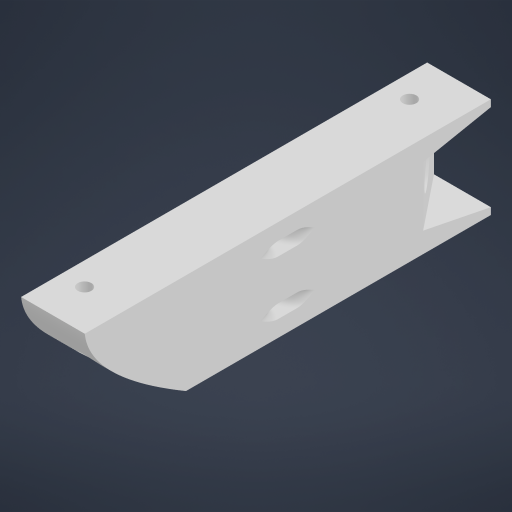
# Autodesk Inventor part: flank
Saved by Autodesk Inventor 2024 (Build 280153000, 153)
## iProperties
Created: 2024-06-07
Part Number: flank
Material: Generic
Document SubType Name: Modeling
Designer: markm
Density: 1 g/cm^3
Appearance: Default
Author: markm
Autodesk Inventor part; units mm, degrees
ref_plane "YZ Plane" through (0, 0, 0) normal (1, 0, 0) x (0, 1, 0)
ref_plane "XZ Plane" through (0, 0, 0) normal (0, 1, 0) x (-1, 0, 0)
sketch "Sketch3" plane through (0, 0, 0) normal (1, 0, 0) x (0, 1, 0)
  line L0 (20, 0) -> (-20, 0)
  line L1 (-20, 0) -> (-20, 150) construction
  line L2 (-20, 150) -> (20, 150) construction
  line L3 (20, 150) -> (20, 0) construction
  line L4 (20, 150) -> (3.094, 150) construction
  line L5 (3.094, 150) -> (-20, 110) construction
  spline S0 degree 2 poles (20, 150) (3.094, 150) (-20, 110) knots 1 1 1 2 2 2
  line L6 (18.5, 149.9225) -> (18.5, 0)
  line L7 (-18.5, 0) -> (-18.5, 112.5669)
  line L8 (0, 0) -> (0, 119.3226) construction
  line L9 (18.5, 0) -> (18.5, 10) construction
  line L10 (18.5, 10) -> (0, 10) construction
  spline S1 degree 2 poles (18.5, 0) (18.5, 10) (0, 10) knots 1 1 1 2 2 2
  line L11 (0, 15) -> (15.8455, 15) construction
  line L12 (-18.5, 0) -> (-18.5, 10) construction
  line L13 (-18.5, 10) -> (0, 10) construction
  spline S2 degree 2 poles (-18.5, 0) (-18.5, 10) (0, 10) knots 1 1 1 2 2 2
  line L14 (16, 0) -> (11, 25)
  line L15 (11, 25) -> (-11, 25)
  line L16 (-11, 25) -> (-16, 0)
  arc A0 (11, 25) -> (-11, 25) centre (0, 22.8) ccw
  dimension "d14" = 40
  dimension "d15" = 150
  dimension "d16" = 40
  dimension "d17" = 30
  dimension "d18" = 1.5
  dimension "d47" = 15
  dimension "d48" = 5
  dimension "d50" = 5
  dimension "d51" = 25
  dimension "d52" = 2.5
  constraints: 22 end point, 9 point on line, 4 perpendicular, 3 horizontal, 3 parallel, 2 point on circle, 1 centre point, 1 coincident, 1 midpoint, 1 symmetric about line, 1 tangent, 13 other
  measures "d14" distance between parallel lines of L1 L3
  measures "d15" distance of L2.end L0.start
  measures "d16" vertical distance of L4.end L5.end
  measures "d17" angle of L1 L5
  measures "d18" distance between parallel lines of L3 L6
  measures "d47" distance between parallel lines of L0 L11
  measures "d48" distance between parallel lines of L11 L10
  measures "d50" horizontal distance of L14.start L14.end
  measures "d51" vertical distance of L14.start L14.end
  measures "d52" distance of L6.end L14.start
extrude "Extrusion3" add sketch "Sketch3" along normal blind 15 and the other way blind 8.5 contours S1 L14 A0 L16 S2 L7 S0 L6 | L0 L14 S1 | L0 S2 L16 | L15 A0
sketch "Sketch4" plane through (-8.5, 18.5, 149.9225) normal (0, 1, 0) x (1, 0, 0)
  line L0 (8.5, 149.9225) -> (8.5, 14.9225) construction
  circle A0 centre (8.5, 14.9225) radius 2.5
  circle A1 centre (8.5, 134.9225) radius 2.5
  line L1 (23.5, 149.9225) -> (23.5, 0) projected
  line L2 (0, 149.9225) -> (23.5, 149.9225) projected
  line L3 (0, 149.9225) -> (11.9483, 138.5432)
  arc A2 (13.5, 134.9225) -> (11.9483, 138.5432) centre (8.5, 134.9225) ccw
  line L4 (13.5, 134.9225) -> (13.5, 99.9225)
  line L5 (13.5, 99.9225) -> (0, 99.9225)
  line L6 (0, 99.9225) -> (0, 149.9225)
  line L7 (2.5, 149.9225) -> (2.5, 99.9225)
  line L8 (0, 0) -> (0, 149.9225) projected
  line L9 (23.5, 124.9225) -> (0, 124.9225)
  line L10 (2.5, 149.9225) -> (23.5, 124.9225)
  point P0 (33.5, 149.9225)
  point P1 (0, 124.9225)
  dimension "d23" = 5
  dimension "d24" = 120
  dimension "d25" = 15
  dimension "d36" = 10
  dimension "d40" = 5
  dimension "d54" = 50
  dimension "d57" = 2.5
  constraints: 16 end point, 5 point on line, 3 centre point, 3 perpendicular, 3 vertical, 2 point on circle, 2 tangent, 1 coincident, 1 concentric, 1 equal radius
  measures "d23" diameter of A0
  measures "d24" distance of A1.centre L0.end
  measures "d25" distance of A1.centre L0.start
  measures "d36" distance of L1.start point (33.5, 149.923)
  measures "d40" radius of A2
  measures "d54" distance between parallel lines of L2 L5
  measures "d57" distance between parallel lines of L6 L7
extrude "Extrusion8" add sketch "Sketch4" against normal up to surface (37 mm away) contours A1 | L9 L4 A2 L3 L7 L10 | L7 L3 L2 | L9 L7 L3 A2 L4 | L3 L7 L9 L6
extrude "Extrusion4" cut sketch "Sketch4" against normal blind 16 contours A0 | A1
sketch "Sketch5" plane through (-8.5, -18.5, 0) normal (0, -1, 0) x (1, 0, 0)
  line L0 (8.5, 0) -> (8.5, 95) construction
  circle A0 centre (8.5, 95) radius 2.5
  circle A1 centre (8.5, 15) radius 2.5
  dimension "d58" = 5
  dimension "d59" = 95
  dimension "d60" = 15
  constraints: 2 centre point, 2 end point, 1 coincident, 1 equal radius, 1 point on line, 1 vertical
  measures "d58" diameter of A1
  measures "d59" distance of L0.start L0.end
  measures "d60" distance of L0.start A1.centre
extrude "Extrusion9" cut sketch "Sketch5" against normal blind 16
sketch "Sketch6" plane through (0, 0, 0) normal (0, 0, 1) x (1, 0, 0)
  arc A0 (3.5291, 0.4815) -> (11.4709, 0.4815) centre (7.5, 0) ccw construction
  circle A1 centre (7.5, 0) radius 5
  line L0 (15, -11) -> (15, 11) construction
  line L1 (15, 0) -> (7.5, 0) construction
  point P0 (0, 0)
  dimension "d63" = 10
  dimension "d69" = 7.5
  constraints: 2 centre point, 2 coincident, 2 end point, 2 point on circle, 1 horizontal, 1 midpoint
  measures "d63" diameter of A1
  measures "d69" distance of L1.start L1.end
extrude "Extrusion10" cut sketch "Sketch6" along normal through all
thicken "Thicken1" [suppressed]
ref_plane "Work Plane1" through (0, 0, 75) normal (0, 0, 1) x (1, 0, 0)
sketch "Sketch8" plane through (0, 0, 75) normal (0, 0, 1) x (1, 0, 0)
  circle A0 centre (7.5, 0) radius 5 construction
  line L0 (-8.5, -18.5) -> (-8.5, 18.5) construction
  line L1 (-8.5, 18.5) -> (15, 18.5) construction
  line L2 (15, 18.5) -> (15, -18.5) construction
  line L3 (15, -18.5) -> (-8.5, -18.5) construction
  line L4 (15, 10) -> (7.5, 10)
  line L5 (-2.5, 0) -> (-2.5, 0)
  line L6 (-2.5, 0) -> (15, 0) construction
  arc A1 (7.5, 10) -> (-2.5, 0) centre (7.5, 0) ccw
  point P0 (0, 0)
  point P1 (-2.5, 10)
  dimension "d71" = 10
  dimension "d72" = 17.5
  dimension "d73" = 10
  constraints: 6 end point, 3 point on line, 2 perpendicular, 2 point on circle, 2 tangent, 1 centre point, 1 horizontal, 1 midpoint
  measures "d71" distance between parallel lines of L6 L4
  measures "d72" distance of L4.start point (-2.5, 10)
  measures "d73" radius of A1
sketch "Sketch9" plane through (15, 0, 0) normal (1, 0, 0) x (0, 0, -1)
  circle A0 centre (-75, 10) radius 2.5
  point P0 (0, 0)
  dimension "d74" = 5
  constraints: 1 centre point, 1 coincident
  measures "d74" diameter of A0
sweep "Sweep1" cut profiles "Sketch9" path "Sketch8" path curves L4 A1
ref_plane "Work Plane2" through (15, 10, 75) normal (0, 1, 0) x (1, 0, 0)
sketch "Sketch10" plane through (15, 10, 75) normal (0, 1, 0) x (1, 0, 0)
  circle A0 centre (-15, -60) radius 2.5 construction
  circle A1 centre (-15, 60) radius 2.5 construction
  line L0 (-21, 75) -> (0, 50) construction
  line L1 (0, 50) -> (0, 2.5) construction
  line L2 (0, 2.5) -> (-7.5, 2.5) construction
  line L3 (-7.5, -2.5) -> (0, -2.5) construction
  line L4 (0, -2.5) -> (0, -71.8354) construction
  line L5 (-23.5, -71.8354) -> (-23.5, 75) construction
  line L6 (-23.5, 75) -> (-21, 75) construction
  arc A2 (0, -10) -> (-7.5, -2.5) centre (-7.5, -10) ccw
  arc A3 (-7.5, 2.5) -> (0, 10) centre (-7.5, 10) ccw
  line L7 (0, 10) -> (0, -10)
  line L8 (-7.5, -2.5) -> (-7.5, 2.5)
  point P0 (-15, 75)
  constraints: 4 end point, 4 point on circle, 2 centre point, 2 point on line, 2 tangent, 1 equal radius, 1 horizontal alignment, 1 vertical, 1 vertical alignment, 1 other
extrude "Extrusion11" cut sketch "Sketch10" along normal mid plane 5
fillet "Fillet1" radius 2.5 4 edges at (12.8033, 12.5, 79.6967) (12.8033, 7.5, 79.6967) (12.8033, 12.5, 70.3033) (12.8033, 7.5, 70.3033)
mirror "Mirror1" about plane through (0, 0, 0) normal (0, 1, 0) of "Sweep1", "Fillet1", "Extrusion11"
body "Solid2"
